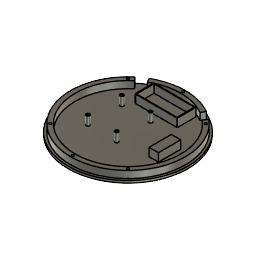
Base_Layer (Autodesk Fusion 360 design; units mm, degrees)
Autodesk Fusion 360 part; units mm, degrees
sketch "Sketch1" plane through (0, 0, 0) normal (0, 0, 1) x (1, 0, 0)
  circle A0 centre (0, 0) radius 102
  dimension "d1" = 204
  constraint coincident A0.centre origin
  measures "d1" diameter of A0
extrude "Extrude1" add sketch "Sketch1" along normal blind 4
sketch "Sketch2" plane through (0, 0, 4) normal (0, 0, 1) x (-1, 0, 0)
  circle A0 centre (0, 0) radius 102
  line L0 (0, 0) -> (0, -98) construction
  circle A1 centre (0, 0) radius 94 construction
  line L1 (0, 0) -> (-49, -84.8705) construction
  line L2 (0, 0) -> (98, 0) construction
  line L3 (0, 0) -> (-62.9932, -75.0724) construction
  line L4 (0, 0) -> (98, 0) construction
  line L5 (0, 0) -> (49, -84.8705) construction
  line L6 (0, 0) -> (98, 0) construction
  line L7 (0, 0) -> (62.9932, -75.0724) construction
  line L8 (0, 0) -> (98, 0) construction
  line L9 (62.9932, -75.0724) -> (57.8509, -68.944)
  line L10 (49, -84.8705) -> (45, -77.9423)
  line L11 (-49, -84.8705) -> (-45, -77.9423)
  line L12 (-62.9932, -75.0724) -> (-57.8509, -68.944)
  arc A2 (62.9932, -75.0724) -> (-62.9932, -75.0724) centre (0, 0) ccw
  arc A3 (-49, -84.8705) -> (49, -84.8705) centre (0, 0) ccw
  arc A4 (57.8509, -68.944) -> (-57.8509, -68.944) centre (0, 0) ccw
  arc A5 (-45, -77.9423) -> (45, -77.9423) centre (0, 0) ccw
  line L13 (0, 0) -> (0, -64) construction
  line L14 (34.5, -79) -> (-34.5, -79)
  line L15 (-34.5, -79) -> (-34.5, -49)
  line L16 (-34.5, -49) -> (34.5, -49)
  line L17 (34.5, -49) -> (34.5, -79)
  line L18 (34.5, -79) -> (-34.5, -49) construction
  line L19 (-34.5, -79) -> (34.5, -49) construction
  line L20 (36, -80) -> (-36, -80)
  line L21 (-36, -80) -> (-36, -48)
  line L22 (-36, -48) -> (36, -48)
  line L23 (36, -48) -> (36, -80)
  line L24 (36, -80) -> (-36, -48) construction
  line L25 (-36, -80) -> (36, -48) construction
  line L26 (0, 0) -> (-63, 0) construction
  line L27 (-55, -19) -> (-71, -19)
  line L28 (-71, -19) -> (-71, 19)
  line L29 (-71, 19) -> (-55, 19)
  line L30 (-55, 19) -> (-55, -19)
  line L31 (-55, -19) -> (-71, 19) construction
  line L32 (-71, -19) -> (-55, 19) construction
  line L33 (0, 0) -> (0, 5) construction
  line L34 (0, 5) -> (20, 5) construction
  line L35 (48, -37.5) -> (-8, -37.5) construction
  line L36 (-8, -37.5) -> (-8, 47.5) construction
  line L37 (-8, 47.5) -> (48, 47.5) construction
  line L38 (48, 47.5) -> (48, -37.5) construction
  line L39 (48, -37.5) -> (-8, 47.5) construction
  line L40 (-8, -37.5) -> (48, 47.5) construction
  line L41 (0, 0) -> (48, -37.5) construction
  line L42 (0, 0) -> (48, 47.5) construction
  line L43 (0, 0) -> (49, 0) construction
  line L44 (0, 0) -> (0, 47.5) construction
  line L45 (0, 0) -> (-8, 47.5) construction
  line L46 (0, 0) -> (-8, 0) construction
  line L47 (0, 0) -> (-8, -37.5) construction
  line L48 (0, 0) -> (-71, -19) construction
  line L49 (0, 0) -> (-71, 19) construction
  circle A6 centre (0, -94) radius 2
  circle A7 centre (0, 94) radius 2
  line L50 (0, 0) -> (66.468, -66.468) construction
  line L51 (0, 0) -> (94, 0) construction
  line L52 (0, 0) -> (-66.468, -66.468) construction
  line L53 (0, 0) -> (94, 0) construction
  circle A8 centre (66.468, -66.468) radius 2 construction
  circle A9 centre (-66.468, -66.468) radius 2 construction
  line L54 (0, 0) -> (-66.468, 66.468) construction
  line L55 (0, 0) -> (94, 0) construction
  circle A10 centre (-66.468, 66.468) radius 2 construction
  line L56 (0, 0) -> (66.468, 66.468) construction
  line L57 (0, 0) -> (94, 0) construction
  circle A11 centre (66.468, 66.468) radius 2 construction
  line L58 (0, 0) -> (24.329, -90.797) construction
  line L59 (0, 0) -> (94, 0) construction
  line L60 (0, 0) -> (-47, 81.4064) construction
  line L61 (0, 0) -> (94, 0) construction
  circle A12 centre (66.468, -66.468) radius 2
  circle A13 centre (-66.468, -66.468) radius 2
  circle A14 centre (66.468, 66.468) radius 2
  circle A15 centre (-66.468, 66.468) radius 2
  point P0 (0, -64)
  point P1 (0, -64)
  point P2 (-63, 0)
  point P3 (20, 5)
  dimension "d4" = 180
  dimension "d5" = 196
  dimension "d6" = 188
  dimension "d7" = 120
  dimension "d8" = 130
  dimension "d9" = 60
  dimension "d10" = 50
  dimension "d11" = 64
  dimension "d12" = 69
  dimension "d13" = 30
  dimension "d14" = 72
  dimension "d15" = 32
  dimension "d16" = 63
  dimension "d17" = 16
  dimension "d18" = 38
  dimension "d19" = 56
  dimension "d20" = 85
  dimension "d21" = 20
  dimension "d22" = 5
  dimension "d23" = 37.999
  dimension "d24" = 44.7
  dimension "d25" = 45.3
  dimension "d26" = 9.56
  dimension "d27" = 14.982
  dimension "d28" = 14.982
  dimension "d29" = 4
  dimension "d30" = 4
  dimension "d31" = 45
  dimension "d32" = 135
  dimension "d33" = 4
  dimension "d34" = 4
  dimension "d35" = 135
  dimension "d36" = 94
  dimension "d37" = 4
  dimension "d38" = 45
  dimension "d39" = 4
  dimension "d40" = 75
  dimension "d41" = 120
  dimension "d42" = 4
  dimension "d43" = 4
  dimension "d44" = 4
  dimension "d45" = 4
  constraint coincident A0.centre L0.start
  constraint concentric A3 A5
  constraint coincident L0.end A3
  constraint vertical L0
  constraint concentric A1 A2
  constraint horizontal L2
  constraint horizontal L4
  constraint horizontal L6
  constraint horizontal L8
  constraint coincident L7 L9.end
  constraint coincident L5 L10.end
  constraint coincident L1 L11.end
  constraint coincident L3 L12.end
  constraint concentric A2 A3
  constraint concentric A4 A5
  constraint parallel L0 L13
  constraint horizontal L14
  constraint perpendicular L14 L15
  constraint parallel L14 L16
  constraint parallel L15 L17
  constraint coincident L18 P1
  constraint coincident L19 P1
  constraint coincident P1 P0
  constraint horizontal L20
  constraint perpendicular L20 L21
  constraint parallel L20 L22
  constraint parallel L21 L23
  constraint coincident L24 P1
  constraint coincident L25 P1
  constraint perpendicular L13 L26
  constraint horizontal L27
  constraint perpendicular L27 L28
  constraint parallel L27 L29
  constraint parallel L28 L30
  constraint coincident L31 P2
  constraint coincident L32 P2
  constraint coincident P2 L26.end
  constraint perpendicular L8 L33
  constraint perpendicular L0 L34
  constraint horizontal L35
  constraint perpendicular L35 L36
  constraint parallel L35 L37
  constraint parallel L36 L38
  constraint coincident L39 P3
  constraint coincident L40 P3
  constraint coincident P3 L34.end
  constraint midpoint L2 L43.end
  constraint perpendicular L43 L44
  constraint coincident L26 L46.end
  constraint coincident L36 L46.end
  constraint coincident A1 A6.centre
  constraint coincident L0 A6.centre
  constraint coincident A1 A7.centre
  constraint horizontal L51
  constraint horizontal L53
  constraint coincident L50.end A8.centre
  constraint coincident L52.end A9.centre
  constraint horizontal L55
  constraint coincident L54.end A10.centre
  constraint horizontal L57
  constraint coincident L56.end A11.centre
  constraint horizontal L59
  constraint horizontal L61
  constraint concentric A8 A12
  constraint concentric A9 A13
  constraint concentric A11 A14
  constraint concentric A10 A15
  measures "d4" diameter of A4
  measures "d5" diameter of A2
  measures "d6" diameter of A1
  measures "d7" angle of L1 L2
  measures "d8" angle of L3 L4
  measures "d9" angle of L5 L6
  measures "d10" angle of L7 L8
  measures "d11" distance of A0.centre P1
  measures "d12" distance of L15.end L16.end
  measures "d13" distance of L14.end L15.end
  measures "d14" distance of L21.end L22.end
  measures "d15" distance of L20.end L21.end
  measures "d16" distance of A0.centre P2
  measures "d17" distance of L28.end L29.end
  measures "d18" distance of L27.end L28.end
  measures "d19" distance of L36.end L37.end
  measures "d20" distance of L35.end L36.end
  measures "d21" distance of L33.end P3
  measures "d22" distance of A0.centre L33.end
  measures "d23" angle of L8 L41
  measures "d24" angle of L2 L42
  measures "d25" angle of L42 L44
  measures "d26" angle of L44 L45
  measures "d27" angle of L26 L48
  measures "d28" angle of L26 L49
  measures "d29" diameter of A6
  measures "d30" diameter of A7
  measures "d31" angle of L50 L51
  measures "d32" angle of L52 L53
  measures "d33" diameter of A8
  measures "d34" diameter of A9
  measures "d35" angle of L54 L55
  measures "d36" distance of A0.centre L54.end
  measures "d37" diameter of A10
  measures "d38" angle of L56 L57
  measures "d39" diameter of A11
  measures "d40" angle of L58 L59
  measures "d41" angle of L60 L61
  measures "d42" diameter of A12
  measures "d43" diameter of A13
  measures "d44" diameter of A14
  measures "d45" diameter of A15
extrude "Extrude2" add sketch "Sketch2" along normal blind 12 contours L9 L12 A2 A4 | L10 L11 A3 A5
sketch "Sketch3" plane through (0, 0, 0) normal (0, 0, -1) x (1, 0, 0)
  circle A0 centre (0, 0) radius 102
  circle A1 centre (0, 0) radius 94 construction
  line L0 (0, 0) -> (-66.468, -66.468) construction
  line L1 (0, 0) -> (94, 0) construction
  line L2 (0, 0) -> (0, -94) construction
  line L3 (0, 0) -> (66.468, -66.468) construction
  line L4 (0, 0) -> (94, 0) construction
  line L5 (0, 0) -> (0, -94) construction
  line L6 (0, 0) -> (66.468, 66.468) construction
  line L7 (0, 0) -> (94, 0) construction
  line L8 (0, 0) -> (0, 94) construction
  line L9 (0, 0) -> (-66.468, 66.468) construction
  line L10 (0, 0) -> (94, 0) construction
  line L11 (150, 0) -> (-200, 0) construction
  circle A2 centre (0, -94) radius 3.75
  circle A3 centre (66.468, -66.468) radius 3.75
  circle A4 centre (-66.468, -66.468) radius 3.75
  circle A5 centre (66.468, 66.468) radius 3.75
  circle A6 centre (0, 94) radius 3.75
  circle A7 centre (-66.468, 66.468) radius 3.75
  dimension "d48" = 188
  dimension "d49" = 135
  dimension "d50" = 45
  dimension "d51" = 45
  dimension "d52" = 135
  dimension "d53" = 7.5
  dimension "d54" = 7.5
  dimension "d55" = 7.5
  constraint concentric A0 A1
  constraint horizontal L1
  constraint coincident A0.centre A1.centre
  constraint coincident A1 L2.end
  constraint perpendicular L1 L2
  constraint horizontal L4
  constraint vertical L5
  constraint horizontal L7
  constraint vertical L8
  constraint horizontal L10
  constraint parallel L10 L11
  constraint coincident L2.end L5.end
  constraint coincident L3.end A3.centre
  constraint coincident L0.end A4.centre
  constraint symmetric L11 A2 A6
  constraint symmetric L11 A3 A5
  constraint symmetric L11 A4 A7
  measures "d48" diameter of A1
  measures "d49" angle of L0 L1
  measures "d50" angle of L3 L4
  measures "d51" angle of L6 L7
  measures "d52" angle of L9 L10
  measures "d53" diameter of A2
  measures "d54" diameter of A3
  measures "d55" diameter of A4
extrude "Extrude3" cut sketch "Sketch3" against normal blind 4.25 contours A2 | A3 | A4 | A5 | A6 | A7
extrude "Extrude4" add sketch "Sketch2" along normal blind 14 contours L20 L21 L22 L23 | L27 L28 L29 L30
sketch "Sketch4" plane through (0, 0, 4) normal (0, 0, 1) x (-1, 0, 0)
  line L0 (-49, -84.8705) -> (-45, -77.9423)
  arc A0 (-45, -77.9423) -> (45, -77.9423) centre (0, 0) ccw
  line L1 (45, -77.9423) -> (49, -84.8705)
  arc A1 (-49, -84.8705) -> (49, -84.8705) centre (0, 0) ccw
  circle A2 centre (0, 0) radius 102
  line L2 (62.9932, -75.0724) -> (57.8509, -68.944)
  arc A3 (57.8509, -68.944) -> (-57.8509, -68.944) centre (0, 0) ccw
  line L3 (-57.8509, -68.944) -> (-62.9932, -75.0724)
  arc A4 (62.9932, -75.0724) -> (-62.9932, -75.0724) centre (0, 0) ccw
  line L4 (-55, 19) -> (-55, -19)
  line L5 (-55, -19) -> (-71, -19)
  line L6 (-71, -19) -> (-71, 19)
  line L7 (-71, 19) -> (-55, 19)
  line L8 (36, -48) -> (36, -80)
  line L9 (36, -80) -> (-36, -80)
  line L10 (-36, -80) -> (-36, -48)
  line L11 (-36, -48) -> (36, -48)
  line L12 (0, 0) -> (0, 5) construction
  line L13 (0, 5) -> (20, 5) construction
  line L14 (48, -37.5) -> (-8, -37.5) construction
  line L15 (-8, -37.5) -> (-8, 47.5) construction
  line L16 (-8, 47.5) -> (48, 47.5) construction
  line L17 (48, 47.5) -> (48, -37.5) construction
  line L18 (48, -37.5) -> (-8, 47.5) construction
  line L19 (-8, -37.5) -> (48, 47.5) construction
  line L20 (20, 47.5) -> (20, -37.5) construction
  line L21 (48, 5) -> (0, 5) construction
  line L22 (48, -37.5) -> (44.5, -37.5) construction
  line L23 (44.5, -37.5) -> (44.5, -34) construction
  line L24 (44.5, -34) -> (44.5, 24) construction
  circle A5 centre (44.5, -34) radius 3
  circle A6 centre (44.5, 24) radius 3
  circle A7 centre (-4.5, -34) radius 3
  circle A8 centre (-4.5, 24) radius 3
  line L25 (-4.5, -34) -> (-4.5, -5) construction
  line L26 (-2, -30) -> (-7, -30) construction
  line L27 (-7, -30) -> (-7, 20) construction
  line L28 (-7, 20) -> (-2, 20) construction
  line L29 (-2, 20) -> (-2, -30) construction
  line L30 (-2, -30) -> (-7, 20) construction
  line L31 (-7, -30) -> (-2, 20) construction
  line L32 (0, 0) -> (0, -5) construction
  line L33 (0, -5) -> (-4.5, -5) construction
  point P0 (20, 5)
  point P1 (-4.5, -5)
  dimension "d60" = 5
  dimension "d61" = 20
  dimension "d62" = 56
  dimension "d63" = 85
  dimension "d64" = 3.5
  dimension "d65" = 3.5
  dimension "d66" = 58
  dimension "d67" = 6
  dimension "d68" = 6
  dimension "d69" = 29
  dimension "d70" = 5
  dimension "d71" = 50
  dimension "d72" = 5
  dimension "d73" = 4.5
  constraint coincident A0.centre A1.centre
  constraint perpendicular L11 L12
  constraint horizontal L13
  constraint horizontal L14
  constraint perpendicular L14 L15
  constraint parallel L14 L16
  constraint parallel L15 L17
  constraint coincident L18 P0
  constraint coincident L19 P0
  constraint coincident P0 L13.end
  constraint midpoint L16 L20.start
  constraint midpoint L14 L20.end
  constraint midpoint L17 L21.start
  constraint perpendicular L17 L22
  constraint perpendicular L22 L23
  constraint parallel L23 L24
  constraint coincident L23.end L24.start
  constraint coincident L24.end A6.centre
  constraint symmetric L20 A5 A7
  constraint symmetric L20 A6 A8
  constraint coincident A7.centre L25.start
  constraint parallel L15 L25
  constraint horizontal L26
  constraint perpendicular L26 L27
  constraint parallel L26 L28
  constraint parallel L27 L29
  constraint coincident L30 P1
  constraint coincident L31 P1
  constraint coincident P1 L25.end
  constraint parallel L12 L32
  measures "d60" distance of A0.centre L12.end
  measures "d61" distance of L12.end P0
  measures "d62" distance of L15.end L16.end
  measures "d63" distance of L14.end L15.end
  measures "d64" distance of L14.start L22.end
  measures "d65" distance of L22.end L23.end
  measures "d66" distance of L23.end L24.end
  measures "d67" diameter of A5
  measures "d68" diameter of A6
  measures "d69" distance of A7.centre P1
  measures "d70" distance of L27.end L28.end
  measures "d71" distance of L26.end L27.end
  measures "d72" distance of A0.centre L32.end
  measures "d73" distance of L32.end P1
extrude "Extrude5" add sketch "Sketch4" along normal blind 15 contours A5 | A6 | A7 | A8
sketch "Sketch5" plane through (0, 0, 19) normal (0, 0, 1) x (-1, 0, 0)
  circle A0 centre (44.5, 24) radius 3
  circle A1 centre (44.5, 24) radius 1.6
  dimension "d76" = 3.2
  constraint concentric A0 A1
  measures "d76" diameter of A1
sketch "Sketch6" plane through (0, 0, 19) normal (0, 0, 1) x (-1, 0, 0)
  circle A0 centre (44.5, -34) radius 3
  circle A1 centre (44.5, -34) radius 1.6
  dimension "d77" = 3.2
  constraint concentric A0 A1
  measures "d77" diameter of A1
sketch "Sketch7" plane through (0, 0, 19) normal (0, 0, 1) x (-1, 0, 0)
  circle A0 centre (-4.5, -34) radius 3
  circle A1 centre (-4.5, -34) radius 1.6
  dimension "d78" = 3.2
  constraint concentric A0 A1
  measures "d78" diameter of A1
sketch "Sketch8" plane through (0, 0, 19) normal (0, 0, 1) x (-1, 0, 0)
  circle A0 centre (-4.5, 24) radius 3
  circle A1 centre (-4.5, 24) radius 1.6
  dimension "d79" = 3.2
  constraint concentric A0 A1
  measures "d79" diameter of A1
extrude "Extrude6" cut sketch "Sketch5" sketch "Sketch7" sketch "Sketch6" sketch "Sketch8" against normal blind 5 contours A1 of sketch 2 contours A1 of sketch 3 contours A1 of sketch 4 contours A1
sketch "Sketch9" plane through (0, 0, 16) normal (0, 0, 1) x (-1, 0, 0)
  circle A0 centre (66.468, -66.468) radius 2
  circle A1 centre (-66.468, 66.468) radius 2
  circle A2 centre (-66.468, -66.468) radius 2
  circle A3 centre (66.468, 66.468) radius 2
  circle A4 centre (0, 94) radius 2
  arc A5 (62.9932, -75.0724) -> (-62.9932, -75.0724) centre (0, 0) ccw
  line L0 (-62.9932, -75.0724) -> (-57.8509, -68.944)
  arc A6 (57.8509, -68.944) -> (-57.8509, -68.944) centre (0, 0) ccw
  line L1 (57.8509, -68.944) -> (62.9932, -75.0724)
  line L2 (0, 0) -> (94, 0) construction
  line L3 (0, 0) -> (94, 0) construction
  constraint horizontal L2
  constraint coincident A5.centre A6.centre
  constraint horizontal L3
